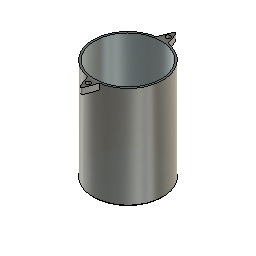
bottom_motor_mag (Autodesk Fusion 360 design; units mm, degrees)
Autodesk Fusion 360 part; units mm, degrees
sketch "Sketch1" plane through (0, 0, 0) normal (0, 0, 1) x (1, 0, 0)
  circle A0 centre (0, 0) radius 29
  dimension "d1" = 58
  constraint coincident A0.centre origin
  measures "d1" diameter of A0
extrude "Extrude1" add sketch "Sketch1" along normal blind 83
extrude "Extrude2" add 1 faces at (-0.5313, 8.3716, 83) along direction (0, 0, 1) blind 2
sketch "Sketch2" plane through (0, 0, 85) normal (0, 0, 1) x (-1, 0, 0)
  circle A0 centre (0, 0) radius 29
  circle A1 centre (0, 0) radius 27.5
  dimension "d6" = 55
  constraint coincident A0.centre A1.centre
  measures "d6" diameter of A1
extrude "Extrude3" cut sketch "Sketch2" against normal blind 83 contours A1
sketch "Sketch3" plane through (0, 0, 0) normal (0, 0, -1) x (1, 0, 0)
  circle A0 centre (0, 0) radius 29
  circle A1 centre (0, 0) radius 15
  dimension "d9" = 30
  constraint coincident A0.centre A1.centre
  measures "d9" diameter of A1
extrude "Extrude4" add sketch "Sketch3" along normal blind 8 contours A1
sketch "Sketch4" plane through (0, 0, -8) normal (0, 0, -1) x (1, 0, 0)
  circle A0 centre (0, 0) radius 15
  circle A1 centre (0, 0) radius 10
  dimension "d12" = 20
  constraint coincident A0.centre A1.centre
  measures "d12" diameter of A1
extrude "Extrude5" add sketch "Sketch4" along normal blind 5 contours A1
sketch "Sketch5" plane through (0, 0, 2) normal (0, 0, 1) x (-1, 0, 0)
  circle A0 centre (0, 0) radius 27.5
sketch "Sketch6" plane through (0, 0, 2) normal (0, 0, 1) x (-1, 0, 0)
  circle A0 centre (0, 0) radius 9
  dimension "d15" = 18
  constraint coincident A0.centre origin
  measures "d15" diameter of A0
extrude "Extrude6" cut sketch "Sketch6" against normal blind 14
sketch "Sketch7" plane through (0, 0, 2) normal (0, 0, 1) x (-1, 0, 0)
  circle A0 centre (0, 0) radius 14
  dimension "d18" = 28
  constraint coincident A0.centre origin
  measures "d18" diameter of A0
extrude "Extrude7" cut sketch "Sketch7" against normal blind 7
fillet "Fillet1" radius 1 1 edges at (-9.3233, 3.6162, -13)
fillet "Fillet2" radius 1 1 edges at (-13.9849, 5.4242, -8)
fillet "Fillet3" radius 1 1 edges at (-27.0375, -10.4868, 0)
sketch "Sketch8" plane through (0, 0, 85) normal (0, 0, 1) x (-1, 0, 0)
  circle A0 centre (0, 0) radius 27.5
  circle A1 centre (0, 0) radius 29
ref_plane "WorkPlane1" through (0, -29, 0) normal (0, 1, 0) x (0, 0, 1)
sketch "Sketch9" plane through (0, 0, 85) normal (0, 0, 1) x (-1, 0, 0)
sketch "Sketch10" plane through (0, 0, 85) normal (0, 0, 1) x (1, 0, 0)
  spline S0 degree 2 poles (5, -28) (0, -43) (-5, -28) knots 0 0 0 2.462214 2.462214 2.462214 weights 1 3 1
  spline S1 degree 2 poles (5, 28) (-0.0113, 43.0942) (-5, 28) knots 0 0 0 2.475135 2.475135 2.475135 weights 1 3 1
  line L0 (5, 28) -> (-5, 28)
  line L1 (5, -28) -> (-5, -28)
  constraint horizontal L0
  constraint parallel L0 L1
extrude "Extrude8" add sketch "Sketch10" against normal blind 5
sketch "Sketch11" plane through (0, 0, 85) normal (0, 0, 1) x (-1, 0, 0)
  circle A0 centre (0, -33.5) radius 1
  dimension "d32" = 2
  measures "d32" diameter of A0
extrude "Extrude9" cut sketch "Sketch11" against normal blind 5
sketch "Sketch12" plane through (0, 0, 85) normal (0, 0, 1) x (-1, 0, 0)
  circle A0 centre (0, -33.5) radius 1
  arc A1 (4.8013, -28.5998) -> (4.7995, 28.6001) centre (0, 0) ccw
  spline S0 degree 2 poles (-4.7995, 28.6001) (0, 42.9309) (4.7995, 28.6001) knots 0.016984 0.016984 0.016984 2.44523 2.44523 2.44523 weights 1.027401 2.972599 1.027401
  arc A2 (-4.7995, 28.6001) -> (-4.8004, -28.5999) centre (0, 0) ccw
  spline S1 degree 2 poles (-4.8004, -28.5999) (0.0113, -43.0251) (4.8013, -28.5998) knots 0.016959 0.016959 0.016959 2.458181 2.458181 2.458181 weights 1.027219 2.972785 1.027211
  circle A3 centre (0, 0) radius 27.5
  circle A4 centre (0, 33) radius 1.9
  dimension "d35" = 3.8
  measures "d35" diameter of A4
extrude "Extrude10" cut sketch "Sketch12" against normal blind 5 contours A4
sketch "Sketch13" plane through (0, 0, 0) normal (0, 0, 1) x (1, 0, 0)
sketch "Sketch14" plane through (0, 0, 85) normal (0, 0, 1) x (-1, 0, 0)
  circle A0 centre (0, 33) radius 1.9
  circle A1 centre (0, -33.5) radius 1
  arc A2 (4.8013, -28.5998) -> (4.7995, 28.6001) centre (0, 0) ccw
  spline S0 degree 2 poles (-4.7995, 28.6001) (0, 42.9309) (4.7995, 28.6001) knots 0.016984 0.016984 0.016984 2.44523 2.44523 2.44523 weights 1.027401 2.972599 1.027401
  arc A3 (-4.7995, 28.6001) -> (-4.8004, -28.5999) centre (0, 0) ccw
  spline S1 degree 2 poles (-4.8004, -28.5999) (0.0113, -43.0251) (4.8013, -28.5998) knots 0.016959 0.016959 0.016959 2.458181 2.458181 2.458181 weights 1.027219 2.972785 1.027211
  circle A4 centre (0, 0) radius 27.5
  circle A5 centre (0, -33.5) radius 1.9
  dimension "d38" = 3.8
  constraint concentric A1 A5
  measures "d38" diameter of A5
extrude "Extrude11" cut sketch "Sketch14" against normal blind 5 contours A5
